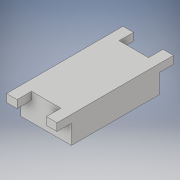
# Autodesk Inventor part: Stamp Body
Saved by Autodesk Inventor 2019.4 (Build 234330000, 330)
## iProperties
Created: 2021-01-06
Part Number: Stamp Body
Material: Generic
Document SubType Name: Modeling
Designer: caleb
Density: 1 g/cm^3
Appearance: Default
Author: caleb
Autodesk Inventor part; units mm, degrees
ref_plane "YZ Plane" through (0, 0, 0) normal (1, 0, 0) x (0, 1, 0)
ref_plane "XZ Plane" through (0, 0, 0) normal (0, 1, 0) x (-1, 0, 0)
ref_plane "XY Plane" through (0, 0, 0) normal (0, 0, 1) x (1, 0, 0)
sketch "Sketch1" plane through (0, 0, 0) normal (0, 1, 0) x (-1, 0, 0)
  line L0 (-13.15, 22.85) -> (13.15, 22.85)
  line L1 (13.15, 22.85) -> (13.15, -22.85)
  line L2 (13.15, -22.85) -> (-13.15, -22.85)
  line L3 (-13.15, -22.85) -> (-13.15, 22.85)
  line L4 (-13.15, 22.85) -> (13.15, -22.85) construction
  line L5 (13.15, 22.85) -> (-13.15, -22.85) construction
  point P0 (0, 0)
  dimension "d0" = 45.7
  dimension "d1" = 26.3
  constraints: 12 end point, 2 midpoint, 2 parallel, 1 horizontal, 1 perpendicular
  measures "d0" distance of L0.end L1.end
  measures "d1" distance of L1.end L2.end
extrude "Extrusion1" add sketch "Sketch1" along normal blind 14
sketch "Sketch2" plane through (0, 14, 0) normal (0, 1, 0) x (1, 0, 0)
  line L0 (-13.15, -22.85) -> (13.15, -22.85) projected
  line L1 (-13.15, -22.85) -> (-7.65, -22.85)
  line L2 (-7.65, -22.85) -> (-7.65, -30.35)
  line L3 (-7.65, -30.35) -> (-13.15, -30.35)
  line L4 (-13.15, -30.35) -> (-13.15, -22.85)
  line L5 (13.15, 22.85) -> (-13.15, 22.85) projected
  line L6 (-13.15, 22.85) -> (-7.65, 22.85)
  line L7 (-7.65, 22.85) -> (-7.65, 30.35)
  line L8 (-7.65, 30.35) -> (-13.15, 30.35)
  line L9 (-13.15, 30.35) -> (-13.15, 22.85)
  line L10 (13.15, 22.85) -> (7.65, 22.85)
  line L11 (7.65, 22.85) -> (7.65, 30.35)
  line L12 (7.65, 30.35) -> (13.15, 30.35)
  line L13 (13.15, 30.35) -> (13.15, 22.85)
  line L14 (13.15, -22.85) -> (13.15, 22.85) projected
  line L15 (13.15, -22.85) -> (7.65, -22.85)
  line L16 (7.65, -22.85) -> (7.65, -30.35)
  line L17 (7.65, -30.35) -> (13.15, -30.35)
  line L18 (13.15, -30.35) -> (13.15, -22.85)
  point P0 (0, 0)
  dimension "d4" = 7.5
  dimension "d5" = 5.5
  constraints: 32 end point, 8 parallel, 4 equal length, 4 horizontal, 4 perpendicular, 2 point on line
  measures "d4" distance of L3.end L0.start
  measures "d5" distance of L2.end L3.end
extrude "Extrusion2" add sketch "Sketch2" against normal blind 4
body "Solid1"
